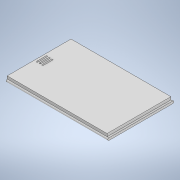
# Autodesk Inventor part: Case-Top
Saved by Autodesk Inventor 2020.2 (Build 242310000, 310)
## iProperties
Created: 2020-03-10
Part Number: Case-Top
Material: Generic
Document SubType Name: Modeling
Designer: dnguy
Density: 1 g/cm^3
Appearance: Default
Author: dnguy
Autodesk Inventor part; units mm, degrees
ref_plane "YZ Plane" through (0, 0, 0) normal (1, 0, 0) x (0, 1, 0)
ref_plane "XZ Plane" through (0, 0, 0) normal (0, 1, 0) x (-1, 0, 0)
ref_plane "XY Plane" through (0, 0, 0) normal (0, 0, 1) x (1, 0, 0)
sketch "Sketch1" plane through (0, 0, 0) normal (1, 0, 0) x (0, 1, 0)
  line L0 (0, 34.5) -> (0, -34.5) construction
  line L1 (-1.25, 34.5) -> (-1.25, -34.5)
  line L2 (1.25, -34.5) -> (1.25, 34.5)
  arc A0 (1.25, 34.5) -> (-1.25, 34.5) centre (0, 34.5) ccw
  arc A1 (-1.25, -34.5) -> (1.25, -34.5) centre (0, -34.5) ccw
  line L3 (0, 0) -> (69, 0) construction
  dimension "d0" = 34.5
  dimension "d1" = 90
  dimension "d2" = 2.5
  constraints: 10 end point, 4 point on circle, 4 tangent, 2 centre point, 1 horizontal, 1 midpoint, 1 parallel, 1 perpendicular, 1 vertical
  measures "d0" distance of L3.start L0.end
  measures "d1" angle of L0 L3
  measures "d2" diameter of A1
sketch "Sketch1 outline for Extrusion1" plane through (0, 0, 0) normal (1, 0, 0) x (0, 1, 0)
  arc A0 (-1.25, -34.5) -> (1.25, -34.5) centre (0, -34.5) ccw
  line L0 (-1.25, 34.5) -> (-1.25, -34.5)
  arc A1 (1.25, 34.5) -> (-1.25, 34.5) centre (0, 34.5) ccw
  line L1 (1.25, -34.5) -> (1.25, 34.5)
extrude "Extrusion1" add sketch "Sketch1 outline for Extrusion1" along normal blind 110
sketch "Sketch2" plane through (0, 1.25, 34.5) normal (0, 1, 0) x (1, 0, 0)
  line L0 (0, 34.5) -> (108, 34.5)
  line L1 (0, 34.5) -> (108, 34.5) construction
  line L2 (108, 34.5) -> (108, 69)
  line L3 (108, 34.5) -> (108, 0)
  line L4 (110, 69) -> (110, 0) projected
  line L5 (108, 34.5) -> (142.5, 34.5) construction
  line L6 (108, 0) -> (108, 69)
  line L7 (108, 69) -> (0, 69)
  line L8 (0, 69) -> (0, 0)
  line L9 (0, 0) -> (108, 0)
  line L10 (110, 69) -> (110, 70.25) projected
  line L11 (0, 69) -> (0, 0) projected
  dimension "d5" = 108
  dimension "d6" = 0
  dimension "d7" = 34.5
  dimension "d8" = 34.5
  dimension "d9" = 90
  constraints: 18 end point, 4 parallel, 3 horizontal, 2 equal length, 2 midpoint, 2 perpendicular
  measures "d5" distance of L0.start L0.end
  measures "d6" distance between parallel lines of L0 L1
  measures "d7" distance of L0.end L2.end
  measures "d8" distance of L1.end L3.end
  measures "d9" angle of L3 L5
sketch "Sketch2 outline for Extrusion2" plane through (0, 1.25, 34.5) normal (0, 1, 0) x (1, 0, 0)
  line L0 (108, 69) -> (0, 69)
  line L1 (108, 34.5) -> (108, 69)
  line L2 (108, 0) -> (108, 34.5)
  line L3 (0, 0) -> (108, 0)
  line L4 (0, 69) -> (0, 0)
extrude "Extrusion2" add sketch "Sketch2 outline for Extrusion2" along normal blind 3
sketch "Sketch3" plane through (0, 4.25, 34.5) normal (0, 1, 0) x (1, 0, 0)
  line L0 (0, 34.5) -> (3, 34.5)
  line L1 (3, 34.5) -> (6, 34.5)
  line L2 (6, 34.5) -> (9, 34.5)
  line L3 (9, 29.5) -> (9, 39.5) construction
  line L4 (9.75, 29.5) -> (9.75, 39.5)
  line L5 (8.25, 39.5) -> (8.25, 29.5)
  arc A0 (8.25, 29.5) -> (9.75, 29.5) centre (9, 29.5) ccw
  arc A1 (9.75, 39.5) -> (8.25, 39.5) centre (9, 39.5) ccw
  line L6 (9, 34.5) -> (19, 34.5) construction
  line L7 (6, 29.5) -> (6, 39.5) construction
  line L8 (6.75, 29.5) -> (6.75, 39.5)
  line L9 (5.25, 39.5) -> (5.25, 29.5)
  arc A2 (5.25, 29.5) -> (6.75, 29.5) centre (6, 29.5) ccw
  arc A3 (6.75, 39.5) -> (5.25, 39.5) centre (6, 39.5) ccw
  line L10 (3, 29.5) -> (3, 39.5) construction
  line L11 (3.75, 29.5) -> (3.75, 39.5)
  line L12 (2.25, 39.5) -> (2.25, 29.5)
  arc A4 (2.25, 29.5) -> (3.75, 29.5) centre (3, 29.5) ccw
  arc A5 (3.75, 39.5) -> (2.25, 39.5) centre (3, 39.5) ccw
  dimension "d12" = 3
  dimension "d13" = 3
  dimension "d14" = 3
  dimension "d15" = 180
  dimension "d16" = 5
  dimension "d17" = 90
  dimension "d18" = 1.5
  dimension "d19" = 5
  dimension "d20" = 1.5
  dimension "d21" = 5
  dimension "d22" = 1.5
  constraints: 32 end point, 12 point on circle, 12 tangent, 6 centre point, 5 equal length, 3 midpoint, 2 horizontal, 2 perpendicular, 1 point on line, 1 vertical
  measures "d12" distance of L0.start L0.end
  measures "d13" distance of L0.end L1.end
  measures "d14" distance of L1.end L2.end
  measures "d15" angle of L2 L1
  measures "d16" distance of L2.end L3.end
  measures "d17" angle of L6 L3
  measures "d18" diameter of A1
  measures "d19" distance of L1.end L7.end
  measures "d20" diameter of A3
  measures "d21" distance of L0.end L10.end
  measures "d22" diameter of A5
sketch "Sketch3 outline for Extrusion3" plane through (0, 4.25, 34.5) normal (0, 1, 0) x (1, 0, 0)
  arc A0 (9.75, 39.5) -> (8.25, 39.5) centre (9, 39.5) ccw
  line L0 (9.75, 29.5) -> (9.75, 39.5)
  arc A1 (8.25, 29.5) -> (9.75, 29.5) centre (9, 29.5) ccw
  line L1 (8.25, 39.5) -> (8.25, 29.5)
  arc A2 (5.25, 29.5) -> (6.75, 29.5) centre (6, 29.5) ccw
  line L2 (5.25, 39.5) -> (5.25, 29.5)
  arc A3 (6.75, 39.5) -> (5.25, 39.5) centre (6, 39.5) ccw
  line L3 (6.75, 29.5) -> (6.75, 39.5)
  arc A4 (2.25, 29.5) -> (3.75, 29.5) centre (3, 29.5) ccw
  line L4 (2.25, 39.5) -> (2.25, 29.5)
  arc A5 (3.75, 39.5) -> (2.25, 39.5) centre (3, 39.5) ccw
  line L5 (3.75, 29.5) -> (3.75, 39.5)
extrude "Extrusion3" add sketch "Sketch3 outline for Extrusion3" along normal blind 2 draft -45
sketch "Sketch4" plane through (0, -1.25, -34.5) normal (0, -1, 0) x (1, 0, 0)
  line L0 (0, 34.5) -> (1.5, 34.5)
  line L1 (1.5, 14.5) -> (1.5, 54.5) construction
  line L2 (6, 39.5) -> (6, 29.5) projected
  line L3 (2.75, 14.5) -> (2.75, 54.5)
  line L4 (0.25, 54.5) -> (0.25, 14.5)
  arc A0 (0.25, 14.5) -> (2.75, 14.5) centre (1.5, 14.5) ccw
  arc A1 (2.75, 54.5) -> (0.25, 54.5) centre (1.5, 54.5) ccw
  line L5 (1.5, 34.5) -> (41.5, 34.5) construction
  dimension "d25" = 1.5
  dimension "d26" = 20
  dimension "d27" = 90
  dimension "d28" = 2.5
  constraints: 12 end point, 4 point on circle, 4 tangent, 2 centre point, 2 horizontal, 2 parallel, 1 midpoint, 1 perpendicular
  measures "d25" distance of L0.start L0.end
  measures "d26" distance of L0.end L1.end
  measures "d27" angle of L5 L1
  measures "d28" diameter of A1
sketch "Sketch4 outline for Extrusion4" plane through (0, -1.25, -34.5) normal (0, -1, 0) x (1, 0, 0)
  arc A0 (2.75, 54.5) -> (0.25, 54.5) centre (1.5, 54.5) ccw
  line L0 (2.75, 14.5) -> (2.75, 54.5)
  arc A1 (0.25, 14.5) -> (2.75, 14.5) centre (1.5, 14.5) ccw
  line L1 (0.25, 54.5) -> (0.25, 14.5)
extrude "Extrusion4" add sketch "Sketch4 outline for Extrusion4" along normal blind 2 draft -45
body "Solid1"
